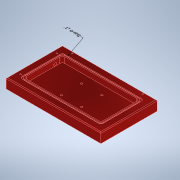
# Autodesk Inventor part: UNLHEP-14-01-P-004_ChuckForGantry
Saved by Autodesk Inventor 2022 (Build 260153000, 153)
## iProperties
Created: 2014-01-09
Part Number: UNLHEP-14-01-P-004_ChuckForGantry
Material: Aluminum, Anodized Red
Document SubType Name: Modeling
Designer: Frank Meier
Density: 2.7 g/cm^3
Project: UNL Pixel Phase I
Mass: 2699.72 g
Surface Area: 1115.91 cm^2
Volume: 999.896 cm^3
Appearance: Anodized - Red
Author: Frank Meier
Revision Number: 00
Autodesk Inventor part; units mm, degrees
ref_plane "YZ Plane" through (0, 0, 0) normal (1, 0, 0) x (0, 1, 0)
ref_plane "XZ Plane" through (0, 0, 0) normal (0, 1, 0) x (-1, 0, 0)
ref_plane "XY Plane" through (0, 0, 0) normal (0, 0, 1) x (1, 0, 0)
sketch "Skizze1" plane through (0, 0, 0) normal (0, 0, 1) x (1, 0, 0)
  line L0 (-117.475, -69.85) -> (117.475, -69.85)
  line L1 (117.475, -69.85) -> (117.475, 69.85)
  line L2 (117.475, 69.85) -> (-117.475, 69.85)
  line L3 (-117.475, 69.85) -> (-117.475, -69.85)
  line L4 (-117.475, -69.85) -> (117.475, 69.85) construction
  line L5 (117.475, -69.85) -> (-117.475, 69.85) construction
  point P0 (0, 0)
  dimension "d0" = 234.95
  dimension "d2" = 139.7
  constraints: 12 end point, 2 midpoint, 2 parallel, 1 horizontal, 1 perpendicular
  measures "d0" distance of L1.end L2.end
  measures "d2" distance of L0.end L1.end
extrude "Extrusion1" add sketch "Skizze1" along normal blind 26
sketch "Skizze2" plane through (0, 0, 26) normal (0, 0, 1) x (1, 0, 0)
  line L0 (-88.9, -47.625) -> (88.9, -47.625)
  line L1 (95.25, -41.275) -> (95.25, 41.275)
  line L2 (88.9, 47.625) -> (-88.9, 47.625)
  line L3 (-95.25, 41.275) -> (-95.25, -41.275)
  line L4 (-95.25, -47.625) -> (95.25, 47.625) construction
  line L5 (95.25, -47.625) -> (-95.25, 47.625) construction
  line L6 (-117.475, -69.85) -> (117.475, -69.85) projected
  line L7 (117.475, -69.85) -> (117.475, 69.85) projected
  line L8 (117.475, 69.85) -> (-117.475, 69.85) projected
  line L9 (-117.475, 69.85) -> (-117.475, -69.85) projected
  circle A0 centre (-109.475, 39.85) radius 2
  circle A1 centre (-87.475, 61.85) radius 2
  circle A2 centre (87.475, 61.85) radius 2
  circle A3 centre (-109.475, -39.85) radius 2
  arc A4 (-88.9, 47.625) -> (-95.25, 41.275) centre (-88.9, 41.275) ccw
  arc A5 (-95.25, -41.275) -> (-88.9, -47.625) centre (-88.9, -41.275) ccw
  arc A6 (88.9, -47.625) -> (95.25, -41.275) centre (88.9, -41.275) ccw
  arc A7 (95.25, 41.275) -> (88.9, 47.625) centre (88.9, 41.275) ccw
  point P0 (0, 0)
  dimension "d5" = 190.5
  dimension "d7" = 95.25
  dimension "d14" = 8
  dimension "d15" = 30
  dimension "d16" = 30
  dimension "d17" = 8
  dimension "d18" = 8
  dimension "d19" = 30
  dimension "d28" = 30
  dimension "d29" = 8
  dimension "d30" = 4
  dimension "d31" = 4
  dimension "d32" = 4
  dimension "d37" = 4
  dimension "d216" = 6.35
  constraints: 12 end point, 8 centre point, 8 point on circle, 8 point on line, 8 tangent, 4 coincident, 3 equal radius, 2 midpoint, 2 parallel, 1 horizontal, 1 perpendicular
  measures "d5" distance of L4.end L5.end
  measures "d7" distance of L5.start L4.end
  measures "d14" distance from line of L9 point (-109.475, 39.85)
  measures "d15" distance from line of L8 point (-109.475, 39.85)
  measures "d16" distance from line of L9 point (-87.475, 61.85)
  measures "d17" distance from line of L8 point (-87.475, 61.85)
  measures "d18" distance from line of L8 point (87.475, 61.85)
  measures "d19" distance from line of L7 point (87.475, 61.85)
  measures "d28" distance from line of L6 point (-109.475, -39.85)
  measures "d29" distance from line of L9 point (-109.475, -39.85)
  measures "d30" diameter of A0
  measures "d31" diameter of A1
  measures "d32" diameter of A2
  measures "d37" diameter of A3
  measures "d216" radius of A4
extrude "Extrusion2" cut sketch "Skizze2" against normal blind 14 contours A5 L3 A4 L2 A7 L1 A6 L0
chamfer "Fase1" distance 2 angle 45 8 edges at (0, -69.85, 26) (-117.475, 0, 26) (0, 69.85, 26) (117.475, 0, 26) (0, -69.85, 0) (-117.475, 0, 0) (0, 69.85, 0) (117.475, 0, 0)
sketch "Skizze4" plane through (0, 0, 26) normal (0, 0, 1) x (1, 0, 0)
  line L0 (117.475, 69.85) -> (-117.475, 69.85) projected
  line L1 (117.475, -69.85) -> (117.475, 69.85) projected
  line L2 (-117.475, 69.85) -> (-117.475, -69.85) projected
  line L3 (-117.475, -69.85) -> (117.475, -69.85) projected
  point P0 (-106.475, 44.85)
  point P1 (-106.475, -44.85)
  point P2 (-87.475, 63.85)
  point P3 (87.475, 63.85)
  dimension "d153" = 25
  dimension "d154" = 25
  dimension "d155" = 11
  dimension "d158" = 11
  dimension "d159" = 6
  dimension "d160" = 30
  dimension "d161" = 30
  dimension "d162" = 6
  measures "d153" distance from line of L0 point (-106.475, 44.85)
  measures "d154" distance from line of L3 point (-106.475, -44.85)
  measures "d155" distance from line of L2 point (-106.475, -44.85)
  measures "d158" distance from line of L2 point (-106.475, 44.85)
  measures "d159" distance from line of L0 point (-87.475, 63.85)
  measures "d160" distance from line of L2 point (-87.475, 63.85)
  measures "d161" distance from line of L1 point (87.475, 63.85)
  measures "d162" distance from line of L0 point (87.475, 63.85)
hole "Bohrung7" at (-87.475, 63.85, 26) at (-106.475, 44.85, 26) at (-106.475, -44.85, 26) at (87.475, 63.85, 26) direction (0, 0, -1) diameter 3.242 depth 20 tip angle 118 thread size "M4x0.7" class "6H" standard "ISO Metric profile"
sketch "Sketch13" plane through (0, 0, 12) normal (0, 0, 1) x (1, 0, 0)
  line L0 (25, -25) -> (-25, -25)
  line L1 (-25, -25) -> (-25, 25)
  line L2 (-25, 25) -> (25, 25)
  line L3 (25, 25) -> (25, -25)
  line L4 (25, -25) -> (-25, 25) construction
  line L5 (-25, -25) -> (25, 25) construction
  point P0 (0, 0)
  dimension "d219" = 50
  dimension "d220" = 50
  constraints: 12 end point, 4 coincident, 2 midpoint, 2 parallel, 1 horizontal, 1 perpendicular
  measures "d219" distance of L1.end L2.end
  measures "d220" distance of L0.end L1.end
hole "Hole9" at (-25, -25, 12) at (25, -25, 12) at (-25, 25, 12) at (25, 25, 12) direction (0, 0, -1) diameter 4.5 end through all clearance for "Flat Head Machine Screw" size "M4" standard "Ansi Metric M Profile"
sketch "Sketch14" plane through (0, 0, 26) normal (0, 0, 1) x (1, 0, 0)
  line L0 (91.44, -50.165) -> (-91.44, -50.165)
  line L1 (-97.79, -43.815) -> (-97.79, 43.815)
  line L2 (-91.44, 50.165) -> (91.44, 50.165)
  line L3 (97.79, 43.815) -> (97.79, -43.815)
  line L4 (97.79, -50.165) -> (-97.79, 50.165) construction
  line L5 (-97.79, -50.165) -> (97.79, 50.165) construction
  line L6 (-88.9, 47.625) -> (88.9, 47.625) projected
  line L7 (95.25, 41.275) -> (95.25, -41.275) projected
  arc A0 (-91.44, 50.165) -> (-97.79, 43.815) centre (-91.44, 43.815) ccw
  arc A1 (-97.79, -43.815) -> (-91.44, -50.165) centre (-91.44, -43.815) ccw
  arc A2 (91.44, -50.165) -> (97.79, -43.815) centre (91.44, -43.815) ccw
  arc A3 (97.79, 43.815) -> (91.44, 50.165) centre (91.44, 43.815) ccw
  line L8 (-94.361, -53.086) -> (94.361, -53.086)
  line L9 (100.711, -46.736) -> (100.711, 46.736)
  line L10 (94.361, 53.086) -> (-94.361, 53.086)
  line L11 (-100.711, 46.736) -> (-100.711, -46.736)
  line L12 (-100.711, -53.086) -> (100.711, 53.086) construction
  line L13 (100.711, -53.086) -> (-100.711, 53.086) construction
  arc A4 (-94.361, 53.086) -> (-100.711, 46.736) centre (-94.361, 46.736) ccw
  arc A5 (-100.711, -46.736) -> (-94.361, -53.086) centre (-94.361, -46.736) ccw
  arc A6 (94.361, -53.086) -> (100.711, -46.736) centre (94.361, -46.736) ccw
  arc A7 (100.711, 46.736) -> (94.361, 53.086) centre (94.361, 46.736) ccw
  point P0 (0, 0)
  dimension "d221" = 2.54
  dimension "d222" = 2.54
  dimension "d223" = 6.35
  dimension "d224" = 2.921
  dimension "d225" = 2.921
  dimension "d226" = 6.35
  constraints: 24 end point, 16 point on circle, 16 point on line, 16 tangent, 8 centre point, 6 equal radius, 4 midpoint, 4 parallel, 2 horizontal, 2 perpendicular
  measures "d221" distance between parallel lines of L2 L6
  measures "d222" distance between parallel lines of L3 L7
  measures "d223" radius of A0
  measures "d224" distance between parallel lines of L10 L2
  measures "d225" distance between parallel lines of L11 L1
  measures "d226" radius of A4
extrude "Extrusion5" cut sketch "Sketch14" against normal blind 2.032
sketch "Sketch15" plane through (-117.475, -69.85, 2) normal (-1, 0, 0) x (0, 0, 1)
  line L0 (-2, 137.7) -> (-2, 2) projected
  line L1 (0, 139.7) -> (22, 139.7) projected
  point P0 (-2, 69.85)
  point P1 (14, 99.7)
  dimension "d230" = 16
  dimension "d231" = 40
  measures "d230" distance from line of L0 point (14, 99.7)
  measures "d231" distance from line of L1 point (14, 99.7)
hole "Hole10" at (-117.475, 29.85, 16) direction (1, 0, 0) diameter 7.9502 depth 22.225 tip angle 118 taper from width 8.7366 to width 8.304 over 6.924 thread size "1/8" designation "1/8 - 27 NPT" standard "NPT"
equation "\"d225\" = d224"
